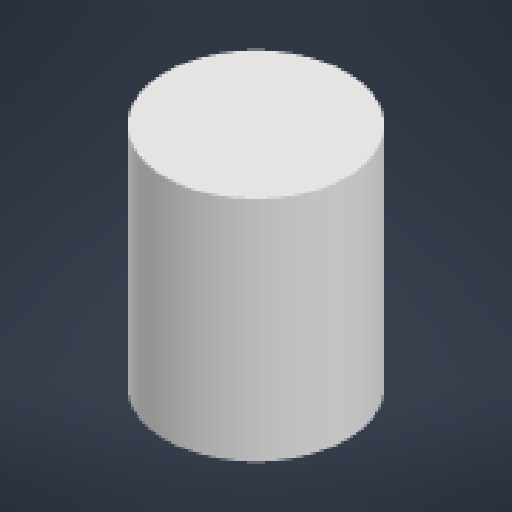
# Autodesk Inventor part: Gear_2
Saved by Autodesk Inventor 2023.4 (Build 274418000, 418)
## iProperties
Created: 2025-10-03
Part Number: Gear_2
Material: Generic
Document SubType Name: Modeling
Designer: Malthe Sennels
Density: 1 g/cm^3
Appearance: Default
Author: Malthe Sennels
Autodesk Inventor part; units mm, degrees
ref_plane "YZ Plane" through (0, 0, 0) normal (1, 0, 0) x (0, 1, 0)
ref_plane "XZ Plane" through (0, 0, 0) normal (0, 1, 0) x (-1, 0, 0)
ref_plane "XY Plane" through (0, 0, 0) normal (0, 0, 1) x (1, 0, 0)
sketch "Sketch1" plane through (0, 0, 0) normal (1, 0, 0) x (0, 1, 0)
  line L0 (51.3905, 30.6355) -> (31.3905, 30.6355)
  line L1 (31.3905, 30.6355) -> (31.3905, 22.6355)
  line L2 (31.3905, 22.6355) -> (51.3905, 22.6355)
  line L3 (51.3905, 22.6355) -> (51.3905, 30.6355)
  point P0 (0, 0)
  dimension "d0" = 20
  dimension "d1" = 8
  constraints: 8 end point, 2 parallel, 1 horizontal, 1 perpendicular
  measures "d0" distance of L2.end L1.end
  measures "d1" distance of L1.end L0.end
revolve "Revolution1" add sketch "Sketch1" angle 360 about axis through (0, 51.3905, 30.6355) along (0, -1, 0)
body "Solid1"
